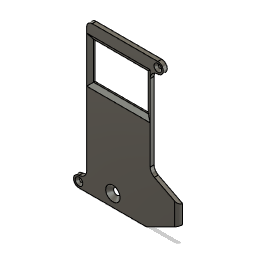
Display cover (Autodesk Fusion 360 design; units mm, degrees)
Autodesk Fusion 360 part; units mm, degrees
sketch "Esboço1" plane through (0, 0, 0) normal (0, 0, 1) x (1, 0, 0)
  line L0 (-0.023, -64.1886) -> (-14.118, -71.2361)
  arc A0 (-15.2361, -71.5) -> (-14.118, -71.2361) centre (-15.2361, -69) ccw
  line L1 (-15.2361, -71.5) -> (-42.5, -71.5)
  line L2 (-42.5, -71.5) -> (-45.5, -71.5)
  arc A1 (-45.5, -66.5) -> (-45.5, -71.5) centre (-45.5, -69) ccw
  arc A2 (-45.5, -66.5) -> (-42, -63) centre (-45.5, -63) ccw
  line L3 (-42, -63) -> (-42, -6)
  arc A3 (-39.5, -3.5) -> (-42, -6) centre (-39.5, -6) ccw
  line L4 (-39.5, -3.5) -> (-13, -3.5)
  line L5 (-9.5001, -3.5) -> (-13, -3.5)
  arc A4 (-9.5501, -8.4995) -> (-9.5001, -3.5) centre (-9.5001, -6) ccw
  line L6 (-9.5501, -8.4995) -> (-9.5966, -8.4995)
  arc A5 (-9.5966, -8.4995) -> (-13.0001, -11.9982) centre (-9.5001, -11.9982) ccw
  line L7 (-13.0001, -11.9982) -> (-13.0001, -47.0056)
  arc A6 (-13.0001, -47.0056) -> (-11.0979, -50.1196) centre (-9.5001, -47.0056) ccw
  line L8 (-11.0979, -50.1196) -> (-0.023, -55.8022)
  line L9 (-0.023, -64.1886) -> (-0.023, -55.8022)
  constraint tangent A6 L8
  constraint tangent A2 L3
  constraint tangent L0 A0
  constraint tangent A3 L4
  constraint tangent A0 L1
  constraint tangent L7 A6
  constraint tangent L2 A1
  constraint tangent L3 A3
  constraint tangent L5 A4
  constraint tangent A5 L7
  constraint vertical L9
extrude "Extrusão1" add sketch "Esboço1" along normal blind 1.8
sketch "Esboço2" plane through (0, 0, 1.8) normal (0, 0, 1) x (1, 0, 0)
  arc A0 (-15.2361, -71.5) -> (-14.118, -71.2361) centre (-15.2361, -69) ccw
  line L0 (-14.118, -71.2361) -> (-0.023, -64.1886)
  line L1 (-0.023, -64.1886) -> (-0.023, -55.8022)
  line L2 (-0.023, -55.8022) -> (-11.0979, -50.1196)
  arc A1 (-13.0001, -47.0056) -> (-11.0979, -50.1196) centre (-9.5001, -47.0056) ccw
  line L3 (-13.0001, -47.0056) -> (-13.0001, -11.9982)
  arc A2 (-9.5966, -8.4995) -> (-13.0001, -11.9982) centre (-9.5001, -11.9982) ccw
  line L4 (-9.5966, -8.4995) -> (-9.5501, -8.4995)
  arc A3 (-9.5501, -8.4995) -> (-9.5001, -3.5) centre (-9.5001, -6) ccw
  line L5 (-9.5001, -3.5) -> (-39.5, -3.5)
  arc A4 (-39.5, -3.5) -> (-42, -6) centre (-39.5, -6) ccw
  line L6 (-42, -6) -> (-42, -63)
  arc A5 (-45.5, -66.5) -> (-42, -63) centre (-45.5, -63) ccw
  arc A6 (-45.5, -66.5) -> (-45.5, -71.5) centre (-45.5, -69) ccw
  line L7 (-45.5, -71.5) -> (-42.5, -71.5)
  line L8 (-42.5, -71.5) -> (-15.2361, -71.5)
  circle A7 centre (-9.5001, -6) radius 0.75
  circle A8 centre (-45.5, -69) radius 0.75
  line L9 (-15.0001, -27.5) -> (-40.0001, -27.5)
  line L10 (-40.0001, -27.5) -> (-40.0001, -10.5)
  line L11 (-40.0001, -10.5) -> (-15.0001, -10.5)
  line L12 (-15.0001, -10.5) -> (-15.0001, -27.5)
  circle A9 centre (-30, -66) radius 1.5
  dimension "d10" = 1.5
  dimension "d11" = 1.5
  dimension "d12" = 25
  dimension "d13" = 17
  dimension "d14" = 2
  dimension "d15" = 1.9999
  dimension "d16" = 7
  dimension "d25" = 3
  constraint concentric A3 A7
  constraint concentric A6 A8
  constraint horizontal L9
  constraint vertical L10
  constraint horizontal L11
  constraint vertical L12
  measures "d10" diameter of A7
  measures "d11" diameter of A8
  measures "d12" distance of L10 L12
  measures "d13" distance of L9 L11
  measures "d14" distance of L3 L12
  measures "d15" distance of L6 L10
  measures "d16" distance of L5 L11
  measures "d25" diameter of A9
extrude "Extrusão2" cut sketch "Esboço2" against normal blind 4 contours A7 | A8 | L9 L10 L11 L12 | A9
chamfer "Chanfro1" distance 1.999 angle 30 4 edges at (-27.5001, -27.5, 1.8) (-40.0001, -19, 1.8) (-27.5001, -10.5, 1.8) (-15.0001, -19, 1.8) measured on face at (-27.7041, -46.3366, 1.8) measured on face at (-27.7041, -46.3366, 1.8) measured on face at (-27.7041, -46.3366, 1.8) measured on face at (-27.7041, -46.3366, 1.8)
fillet "Arredondamento1" radius 1.8 1 edges at (-0.023, -59.9954, 1.8)
chamfer "Chanfro2" distance 1 angle 45 2 edges at (-10.1993, -5.7288, 1.8) (-46.1992, -68.7288, 1.8) measured on face at (-28.3704, -47.0029, 1.8) measured on face at (-28.3704, -47.0029, 1.8)
chamfer "Chanfro3" distance 1.8 angle 45 1 edges at (-31.3985, -65.4576, 1.8) measured on face at (-28.3704, -47.0029, 1.8)
